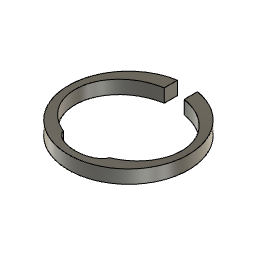
anchor_ring v3 (Autodesk Fusion 360 design; units mm, degrees)
Autodesk Fusion 360 part; units mm, degrees
sketch "Sketch1" plane through (0, 0, 0) normal (0, 0, 1) x (1, 0, 0)
  line L0 (1.5, 6.8374) -> (1.5, 8.8741)
  line L1 (-1.5, 8.8741) -> (-1.5, 6.8374)
  line L2 (-10.5245, 0) -> (10.5245, 0)
  arc A0 (-1.5, 8.8741) -> (1.5, 8.8741) centre (0, 0) ccw
  line L3 (0, 8.6614) -> (0, -8.6614) construction
  ellipse E0 centre (0, 0) end of major axis (8, 0) minor radius 7
  line L4 (-8, 0) -> (8, 0)
  line L5 (0, -7) -> (0, 7)
  dimension "d2" = 18
  dimension "d5" = 3
  dimension "d30" = 16
  dimension "d31" = 14
  constraint coincident A0.centre E0.centre
  constraint vertical L0
  constraint vertical L1
  constraint perpendicular L1 L2
  constraint perpendicular L2 L3
  constraint symmetric L0 L1 L3
  constraint midpoint A0.centre L3
  constraint midpoint A0.centre L2
  constraint coincident E0 L4.start
  constraint coincident E0 L4.end
  constraint coincident E0 L5.start
  constraint coincident E0 L5.end
  constraint perpendicular L3 L4
  measures "d2" diameter of A0
  measures "d5" distance of L0 L1
  measures "d30" distance of E0
extrude "Extrude6" add sketch "Sketch1" along normal blind 2 contours L0 L2 A0 E0 | L2 A0 E0 | L1 L2 A0 E0
sketch "Sketch2" plane through (0, 0, 0) normal (0, 1, 0) x (1, 0, 0)
sketch "Sketch3" plane through (0, 0, 2) normal (0, 0, 1) x (-1, 0, 0)
  arc A0 (-9, 0) -> (-1.5, -8.8741) centre (0, 0) ccw
  line L0 (-1.5, -8.8741) -> (-1.5, -6.8759)
  line L1 (7.8349, 0) -> (-7.8349, 0)
  line L2 (0, -10.7948) -> (0, 10.7948)
  ellipse E0 centre (0, 6) end of major axis (-6, 6) minor radius 3
  line L3 (6, 6) -> (-6.1851, 6)
  line L4 (0, 9) -> (0, 3)
  ellipse E1 centre (0, 6) end of major axis (-3.5, 6) minor radius 2
  line L5 (3.5, 6) -> (-3.5, 6)
  line L6 (0, 8) -> (0, 4)
  ellipse E2 centre (0, 0) end of major axis (-8, 0) minor radius 7 (-8, 0) -> (-1.5, -6.8759) ccw
  line L7 (-8, 0) -> (-9, 0)
  dimension "d15" = 12
  dimension "d16" = 6
  dimension "d17" = 7
  dimension "d18" = 4
  constraint horizontal L1
  constraint vertical L2
  constraint midpoint L1 A0.centre
  constraint midpoint L2 A0.centre
  constraint coincident E0 L3.start
  constraint coincident E0 L4.start
  constraint coincident E0 L4.end
  constraint coincident L2 E0.centre
  constraint coincident E1 L5.start
  constraint coincident E1 L5.end
  constraint coincident E1 L6.start
  constraint coincident E1 L6.end
  constraint concentric E0 E1
  constraint collinear L3 L5
  measures "d15" distance of E0
  measures "d16" distance of E0
  measures "d17" distance of E1
extrude "Extrude7" cut sketch "Sketch3" against normal up to surface (2 mm away) contours L2 L3 L4 E1 L5 L6 | L2 L3 L4 E1 L5 L6 | L2 L3 L4 E1 L5 L6 | L2 L3 L4 E1 L5 L6
extrude "Extrude2" [suppressed]
extrude "Extrude3" [suppressed]
extrude "Extrude4" [suppressed]
extrude "Extrude5" [suppressed]
